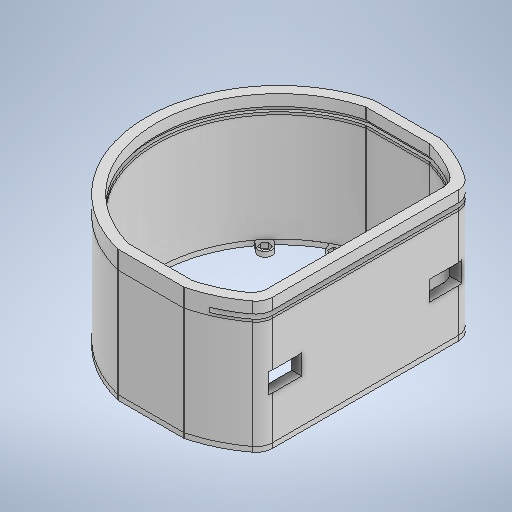
# Autodesk Inventor part: carcasa4.0
Saved by Autodesk Inventor 2025.3 (Build 293356030, 356C)
## iProperties
Created: 2025-08-27
Part Number: carcasa4.0
Material: Generic
Document SubType Name: Modeling
Designer: cdavi
Density: 1 g/cm^3
Appearance: Default
Author: cdavi
Autodesk Inventor part; units mm, degrees
ref_plane "YZ Plane" through (0, 0, 0) normal (1, 0, 0) x (0, 1, 0)
ref_plane "XZ Plane" through (0, 0, 0) normal (0, 1, 0) x (-1, 0, 0)
ref_plane "XY Plane" through (0, 0, 0) normal (0, 0, 1) x (1, 0, 0)
sketch "Sketch1" plane through (0, 0, 0) normal (0, 1, 0) x (-1, 0, 0)
  line L0 (18.8082, 71.5) -> (-18.8082, 71.5)
  line L1 (0, 0) -> (-52, 0) construction
  line L2 (19.5895, 77.5) -> (-19.5895, 77.5)
  line L3 (18.8082, -71.5) -> (-19.0722, -71.5)
  line L4 (19.5895, -77.5) -> (-19.5895, -77.5)
  line L5 (0, 0) -> (0, 77.5) construction
  line L6 (-46, 52.915) -> (-46, -52.915)
  line L7 (-52, 56) -> (-52, -56)
  arc A0 (-41.625, -61.183) -> (-19.0722, -71.5) centre (0, 0) ccw
  arc A1 (-48, -64) -> (-20.0918, -77.4359) centre (0, 0) ccw
  arc A2 (20.0918, -77.4359) -> (20.0918, 77.4359) centre (0, 0) ccw
  arc A3 (-20.0918, 77.4359) -> (-48, 64) centre (0, 0) ccw
  arc A4 (19.3307, -71.4306) -> (19.3307, 71.4306) centre (0, 0) ccw
  arc A5 (-19.3307, 71.4306) -> (-41.625, 61.183) centre (0, 0) ccw
  arc A6 (-20.0918, -77.4359) -> (-19.5895, -77.5) centre (-19.5895, -75.5) ccw
  arc A7 (19.5895, -77.5) -> (20.0918, -77.4359) centre (19.5895, -75.5) ccw
  arc A8 (18.8082, -71.5) -> (19.3307, -71.4306) centre (18.8082, -69.5) ccw
  arc A9 (19.3307, 71.4306) -> (18.8082, 71.5) centre (18.8082, 69.5) ccw
  arc A10 (20.0918, 77.4359) -> (19.5895, 77.5) centre (19.5895, 75.5) ccw
  arc A11 (-18.8082, 71.5) -> (-19.3307, 71.4306) centre (-18.8082, 69.5) ccw
  arc A12 (-19.5895, 77.5) -> (-20.0918, 77.4359) centre (-19.5895, 75.5) ccw
  arc A13 (-41.625, 61.183) -> (-46, 52.915) centre (-36, 52.915) ccw
  arc A14 (-48, 64) -> (-52, 56) centre (-42, 56) ccw
  arc A15 (-52, -56) -> (-48, -64) centre (-42, -56) ccw
  arc A16 (-46, -52.915) -> (-41.625, -61.183) centre (-36, -52.915) ccw
  point P0 (-19.8431, 77.5)
  point P1 (19.0722, -71.5)
  point P2 (19.8431, -77.5)
  point P3 (-19.8431, -77.5)
  point P4 (-52, -60.7947)
  point P5 (-46, 57.9655)
  point P6 (-46, -57.9655)
  point P7 (-52, 60.7947)
  point P8 (19.8431, 77.5)
  point P9 (19.0722, 71.5)
  point P10 (-19.0722, 71.5)
  dimension "d2" = 71.5
  dimension "d4" = 6
  dimension "d6" = 46
  dimension "d7" = 6
  dimension "d8" = 2
  dimension "d9" = 10
  dimension "d10" = 74
  dimension "d11" = 80
  dimension "d12" = 74
  dimension "d13" = 80
  constraints: 45 point on circle, 22 tangent, 17 centre point, 16 end point, 11 point on line, 9 equal radius, 4 symmetric about line, 3 vertical, 2 coincident, 2 horizontal, 2 midpoint, 1 parallel
  measures "d2" distance between parallel lines of L1 L0
  measures "d4" distance between parallel lines of L0 L2
  measures "d6" distance between parallel lines of L6 L5
  measures "d7" distance between parallel lines of L7 L6
  measures "d8" radius of A6
  measures "d9" radius of A13
  measures "d10" radius of A4
  measures "d11" radius of A2
  measures "d12" radius of A0
  measures "d13" radius of A1
extrude "Extrusion1" add sketch "Sketch1" along normal blind 65
sketch "Sketch2" plane through (52, 0, 56) normal (1, 0, 0) x (0, 0, -1)
  line L0 (56, 0) -> (56, 65) construction
  line L1 (108.915, 65) -> (3.085, 65) projected
  line L2 (-2.4359, 38) -> (17.5641, 38)
  line L3 (17.5641, 38) -> (17.5641, 26)
  line L4 (17.5641, 26) -> (-2.4359, 26)
  line L5 (-2.4359, 26) -> (-2.4359, 38)
  line L6 (0, 0) -> (112, 0) projected
  line L7 (-21.4359, 0) -> (-21.4359, 65) projected
  line L8 (114.4359, 38) -> (94.4359, 38)
  line L9 (94.4359, 38) -> (94.4359, 26)
  line L10 (94.4359, 26) -> (114.4359, 26)
  line L11 (114.4359, 26) -> (114.4359, 38)
  dimension "d16" = 26
  dimension "d17" = 19
  dimension "d18" = 12
  dimension "d19" = 20
  constraints: 18 end point, 4 symmetric about line, 2 parallel, 1 horizontal, 1 midpoint, 1 perpendicular
  measures "d16" distance between parallel lines of L6 L4
  measures "d17" distance between parallel lines of L5 L7
  measures "d18" distance of L2.end L3.end
  measures "d19" distance of L2.start L2.end
extrude "Extrusion2" cut sketch "Sketch2" against normal blind 13.25
sketch "Sketch3" plane through (52, 0, 56) normal (1, 0, 0) x (0, 0, -1)
  line L0 (3.568, 49.2223) -> (17.7975, 43.9952) construction
  line L1 (2.8909, 47.379) -> (17.1204, 42.1519)
  line L2 (18.4746, 45.8385) -> (4.2452, 51.0656)
  arc A0 (4.2452, 51.0656) -> (2.8909, 47.379) centre (3.568, 49.2223) ccw
  arc A1 (17.1204, 42.1519) -> (18.4746, 45.8385) centre (17.7975, 43.9952) ccw
  arc A2 (44.4296, 11.624) -> (34.6921, 2.9774) centre (43.8866, 2.4292) ccw construction
  arc A3 (44.531, 13.3402) -> (32.9759, 3.0797) centre (43.8866, 2.4292) ccw
  arc A4 (44.3283, 9.9077) -> (36.4083, 2.8751) centre (43.8866, 2.4292) ccw
  arc A5 (44.3283, 9.9077) -> (44.531, 13.3402) centre (44.4296, 11.624) ccw
  arc A6 (32.9759, 3.0797) -> (36.4083, 2.8751) centre (34.6921, 2.9774) ccw
  line L3 (56, 0) -> (56, 65) construction
  line L4 (109.1091, 47.379) -> (94.8796, 42.1519)
  line L5 (93.5254, 45.8385) -> (107.7548, 51.0656)
  arc A7 (109.1091, 47.379) -> (107.7548, 51.0656) centre (108.432, 49.2223) ccw
  arc A8 (93.5254, 45.8385) -> (94.8796, 42.1519) centre (94.2025, 43.9952) ccw
  point P0 (10.6828, 46.6088)
  constraints: 18 point on circle, 12 end point, 9 centre point, 8 tangent, 6 symmetric about line, 1 midpoint, 1 parallel, 2 other
extrude "Extrusion3" [suppressed]
extrude "Extrusion4" add sketch "Sketch1" along normal blind 3 from surface at 65 separate body contours A9 A4 A8 L3 A0 A16 L6 A13 A5 A11 L0 | A10 A2 A7 L4 A6 A1 A15 L7 A14 A3 A12 L2
sketch "Sketch5" plane through (-19.5895, 68, 77.5) normal (0, 1, 0) x (1, 0, 0)
  circle A0 centre (19.5895, 77.5) radius 8.5
  circle A1 centre (-10.4105, 77.5) radius 2.5
  line L0 (27.7136, 75) -> (36.5895, 75)
  line L1 (36.5895, 75) -> (36.5895, 80)
  line L2 (36.5895, 80) -> (27.7136, 80)
  line L3 (36.5895, 77.5) -> (71.5895, 77.5)
  line L4 (71.5895, 21.5) -> (71.5895, 133.5) projected
  line L5 (-10.4105, 77.5) -> (-60.4105, 77.5)
  arc A2 (-0.5023, 154.9359) -> (-0.5023, 0.0641) centre (19.5895, 77.5) ccw projected
  dimension "d26" = 17
  dimension "d27" = 5
  dimension "d31" = 5
  dimension "d32" = 17
  dimension "d47" = 30
  dimension "d204" = 35
  dimension "d205" = 50
  dimension "d206" = 52
  constraints: 10 end point, 3 point on circle, 2 centre point, 2 horizontal alignment, 2 midpoint, 2 perpendicular, 1 coincident, 1 horizontal, 1 point on line
  measures "d26" diameter of A0
  measures "d27" diameter of A1
  measures "d31" distance between parallel lines of L2 L0
  measures "d32" distance from line of A0.centre L1
  measures "d47" distance of A0.centre L5.start
  measures "d204" distance of L3.start L3.end
  measures "d205" distance of L5.start L5.end
  measures "d206" distance from line of L4 point (19.59, 77.5)
extrude "Extrusion5" cut sketch "Sketch5" against normal through all bodies 2
sketch "Sketch6" plane through (0, 0, 0) normal (0, 1, 0) x (-1, 0, 0)
  circle A0 centre (0, 0) radius 69 construction
  arc A1 (-19.3307, 71.4306) -> (-41.625, 61.183) centre (0, 0) ccw projected
  arc A2 (-41.625, 61.183) -> (-46, 52.915) centre (-36, 52.915) ccw projected
  line L0 (-46, -52.915) -> (-46, 52.915) projected
  arc A3 (-46, -52.915) -> (-41.625, -61.183) centre (-36, -52.915) ccw projected
  arc A4 (-41.625, -61.183) -> (-19.0722, -71.5) centre (0, 0) ccw projected
  line L1 (18.8082, -71.5) -> (-19.0722, -71.5) construction
  arc A5 (19.3307, -71.4306) -> (19.3307, 71.4306) centre (0, 0) ccw projected
  line L2 (-18.8082, 71.5) -> (18.8082, 71.5) construction
  line L3 (19.5895, 77.5) -> (-19.5895, 77.5) projected
  arc A6 (-20.0918, 77.4359) -> (-48, 64) centre (0, 0) ccw projected
  arc A7 (-48, 64) -> (-52, 56) centre (-42, 56) ccw projected
  line L4 (-52, 56) -> (-52, -56) projected
  arc A8 (-52, -56) -> (-48, -64) centre (-42, -56) ccw projected
  arc A9 (-48, -64) -> (-20.0918, -77.4359) centre (0, 0) ccw projected
  line L5 (-19.5895, -77.5) -> (19.5895, -77.5) projected
  arc A10 (20.0918, -77.4359) -> (20.0918, 77.4359) centre (0, 0) ccw projected
  arc A11 (-18.5383, 65.4242) -> (-38.25, 56.2222) centre (0, 0) ccw construction
  arc A12 (-38.25, 56.2222) -> (-40, 52.915) centre (-36, 52.915) ccw construction
  line L6 (-40, 52.915) -> (-40, -52.915) construction
  arc A13 (-40, -52.915) -> (-38.25, -56.2222) centre (-36, -52.915) ccw construction
  arc A14 (-38.25, -56.2222) -> (-18.5383, -65.4242) centre (0, 0) ccw construction
  line L7 (-17.9931, -65.5) -> (17.9931, -65.5) construction
  line L8 (-17.9931, 65.5) -> (17.9931, 65.5) construction
  arc A15 (18.5383, -65.4242) -> (18.5383, 65.4242) centre (0, 0) ccw construction
  arc A16 (-8.124, -2.5) -> (-8.124, 2.5) centre (0, 0) ccw projected
  line L9 (0, 0) -> (52.8571, 44.3523) construction
  line L10 (0, 0) -> (80, 0) construction
  circle A17 centre (52.8571, 44.3523) radius 3.1 construction
  line L11 (0, 0) -> (0, -69) construction
  circle A18 centre (29.1607, 62.5352) radius 3.1 construction
  line L12 (29.1607, 62.5352) -> (0, 0) construction
  circle A19 centre (-42.5, 20) radius 3.1 construction
  circle A20 centre (-29.1607, 62.5352) radius 3.1 construction
  line L13 (-29.1607, 62.5352) -> (0, 0) construction
  arc A21 (-17.9931, 65.5) -> (-18.5383, 65.4242) centre (-17.9931, 63.5) ccw construction
  arc A22 (-18.5383, -65.4242) -> (-17.9931, -65.5) centre (-17.9931, -63.5) ccw construction
  arc A23 (17.9931, -65.5) -> (18.5383, -65.4242) centre (17.9931, -63.5) ccw construction
  arc A24 (18.5383, 65.4242) -> (17.9931, 65.5) centre (17.9931, 63.5) ccw construction
  arc A25 (-20.0918, -77.4359) -> (-19.5895, -77.5) centre (-19.5895, -75.5) ccw projected
  arc A26 (19.5895, -77.5) -> (20.0918, -77.4359) centre (19.5895, -75.5) ccw projected
  arc A27 (20.0918, 77.4359) -> (19.5895, 77.5) centre (19.5895, 75.5) ccw projected
  arc A28 (-19.5895, 77.5) -> (-20.0918, 77.4359) centre (-19.5895, 75.5) ccw projected
  circle A29 centre (52.8571, -44.3523) radius 3.1 construction
  circle A30 centre (29.1607, -62.5352) radius 3.1 construction
  circle A31 centre (-42.5, -20) radius 3.1 construction
  circle A32 centre (-29.1607, -62.5352) radius 3.1 construction
  line L14 (19.3307, 65.1945) -> (19.3307, 71.4306)
  line L15 (-19.3307, 65.1945) -> (-19.3307, 71.4306)
  line L16 (19.3307, 71.4306) -> (-19.3307, 71.4306)
  line L17 (19.3307, -65.1945) -> (19.3307, -71.4306)
  line L18 (-19.3307, -65.1945) -> (-19.3307, -71.4306)
  line L19 (19.3307, -71.4306) -> (-19.3307, -71.4306)
  circle A33 centre (52.8571, 44.3523) radius 4
  circle A34 centre (29.1607, 62.5352) radius 4
  line L20 (49.8042, 43.814) -> (50.8644, 46.7271)
  line L21 (50.8644, 46.7271) -> (53.9173, 47.2654)
  line L22 (53.9173, 47.2654) -> (55.91, 44.8907)
  line L23 (55.91, 44.8907) -> (54.8497, 41.9776)
  line L24 (54.8497, 41.9776) -> (51.7968, 41.4393)
  line L25 (51.7968, 41.4393) -> (49.8042, 43.814)
  line L26 (26.6213, 60.7572) -> (26.3511, 63.8454)
  line L27 (26.3511, 63.8454) -> (28.8905, 65.6234)
  line L28 (28.8905, 65.6234) -> (31.7, 64.3133)
  line L29 (31.7, 64.3133) -> (31.9702, 61.2251)
  line L30 (31.9702, 61.2251) -> (29.4308, 59.447)
  line L31 (29.4308, 59.447) -> (26.6213, 60.7572)
  circle A35 centre (-42.5, 20) radius 4
  line L32 (-45.1847, 18.45) -> (-45.1847, 21.55)
  line L33 (-45.1847, 21.55) -> (-42.5, 23.1)
  line L34 (-42.5, 23.1) -> (-39.8153, 21.55)
  line L35 (-39.8153, 21.55) -> (-39.8153, 18.45)
  line L36 (-39.8153, 18.45) -> (-42.5, 16.9)
  line L37 (-42.5, 16.9) -> (-45.1847, 18.45)
  line L38 (-42.5, 24) -> (-46, 24)
  line L39 (-42.5, 16) -> (-46, 16)
  circle A36 centre (-29.1607, 62.5352) radius 4
  line L40 (-29.4308, 59.447) -> (-31.9702, 61.2251)
  line L41 (-31.9702, 61.2251) -> (-31.7, 64.3133)
  line L42 (-31.7, 64.3133) -> (-28.8905, 65.6234)
  line L43 (-28.8905, 65.6234) -> (-26.3511, 63.8454)
  line L44 (-26.3511, 63.8454) -> (-26.6213, 60.7572)
  line L45 (-26.6213, 60.7572) -> (-29.4308, 59.447)
  line L46 (-32.7354, 60.7404) -> (-34.9798, 65.2105)
  circle A37 centre (52.8571, -44.3523) radius 4
  circle A38 centre (29.1607, -62.5352) radius 4
  circle A39 centre (-42.5, -20) radius 4
  line L47 (-42.5, -24) -> (-46, -24)
  line L48 (-42.5, -16) -> (-46, -16)
  circle A40 centre (-29.1607, -62.5352) radius 4
  line L49 (-32.7354, -60.7404) -> (-34.9798, -65.2105)
  line L50 (49.8042, -43.814) -> (50.8644, -46.7271)
  line L51 (50.8644, -46.7271) -> (53.9173, -47.2654)
  line L52 (53.9173, -47.2654) -> (55.91, -44.8907)
  line L53 (55.91, -44.8907) -> (54.8497, -41.9776)
  line L54 (54.8497, -41.9776) -> (51.7968, -41.4393)
  line L55 (51.7968, -41.4393) -> (49.8042, -43.814)
  line L56 (26.6213, -60.7572) -> (26.3511, -63.8454)
  line L57 (26.3511, -63.8454) -> (28.8905, -65.6234)
  line L58 (28.8905, -65.6234) -> (31.7, -64.3133)
  line L59 (31.7, -64.3133) -> (31.9702, -61.2251)
  line L60 (31.9702, -61.2251) -> (29.4308, -59.447)
  line L61 (29.4308, -59.447) -> (26.6213, -60.7572)
  line L62 (-29.4308, -59.447) -> (-31.9702, -61.2251)
  line L63 (-31.9702, -61.2251) -> (-31.7, -64.3133)
  line L64 (-31.7, -64.3133) -> (-28.8905, -65.6234)
  line L65 (-28.8905, -65.6234) -> (-26.3511, -63.8454)
  line L66 (-26.3511, -63.8454) -> (-26.6213, -60.7572)
  line L67 (-26.6213, -60.7572) -> (-29.4308, -59.447)
  line L68 (-45.1847, -18.45) -> (-45.1847, -21.55)
  line L69 (-45.1847, -21.55) -> (-42.5, -23.1)
  line L70 (-42.5, -23.1) -> (-39.8153, -21.55)
  line L71 (-39.8153, -21.55) -> (-39.8153, -18.45)
  line L72 (-39.8153, -18.45) -> (-42.5, -16.9)
  line L73 (-42.5, -16.9) -> (-45.1847, -18.45)
  line L74 (50.1982, 47.3407) -> (53.9351, 50.6656)
  line L75 (55.3383, 41.2149) -> (59.2616, 44.3177)
  line L76 (32.7354, 60.7404) -> (34.9798, 65.2105)
  line L77 (50.1982, -47.3407) -> (53.9351, -50.6656)
  line L78 (55.3383, -41.2149) -> (59.2616, -44.3177)
  line L79 (32.7354, -60.7404) -> (34.9798, -65.2105)
  line L80 (-25.488, 64.1199) -> (-27.4696, 68.7126)
  line L81 (25.488, 64.1199) -> (27.4696, 68.7126)
  line L82 (-25.488, -64.1199) -> (-27.4696, -68.7126)
  line L83 (25.488, -64.1199) -> (27.4696, -68.7126)
  line L84 (-18.8082, 71.5) -> (-52, 71.5)
  line L85 (-52, 71.5) -> (-52, 56)
  line L86 (-35.8852, 71.5) -> (-18.8082, 71.5)
  point P0 (-18.2688, -65.5)
  point P1 (-19.3307, 65.1945)
  point P2 (-19.3307, -65.1945)
  point P3 (29.1607, 62.5352)
  point P4 (-19.3307, -71.4306)
  point P5 (-34.9798, -65.2105)
  point P6 (-46, -24)
  point P7 (-46, -16)
  point P8 (59.2616, -44.3177)
  point P9 (55.3383, -41.2149)
  point P10 (34.9798, -65.2105)
  point P11 (-27.9581, 66.3502)
  point P12 (-27.9581, -66.3502)
  point P13 (27.9581, -66.3502)
  point P14 (27.9581, 66.3502)
  point P15 (-46, 21.9365)
  point P16 (-46, 18.0635)
  point P17 (-32.8561, 64.0662)
  point P18 (32.8561, -64.0662)
  point P19 (56.8533, -44.1781)
  point P20 (53.3794, -48.3181)
  point P21 (-32.8561, -64.0662)
  point P22 (-46, -21.9365)
  point P23 (-46, -18.0635)
  point P24 (53.3794, 48.3181)
  point P25 (56.8533, 44.1781)
  point P26 (32.8561, 64.0662)
  point P27 (25.488, -64.1199)
  point P28 (27.4696, -68.7126)
  point P29 (-25.488, -64.1199)
  point P30 (34.0084, -67.0387)
  point P31 (-28.5882, -71.3052)
  point P32 (28.5882, -71.3052)
  point P33 (28.5882, 71.3052)
  point P34 (-28.5882, 71.3052)
  point P35 (34.0084, 67.0387)
  point P36 (-19.3307, -71.4306)
  point P37 (-34.0084, -67.0387)
  point P38 (-34.0084, 67.0387)
  dimension "d33" = 138
  dimension "d39" = 6.2
  dimension "d34" = 6
  dimension "d35" = 6
  dimension "d36" = 6
  dimension "d37" = 40
  dimension "d38" = 25
  dimension "d40" = 20
  dimension "d41" = 3.5
  dimension "d42" = 25
  dimension "d44" = 2
  dimension "d61" = 8
  dimension "d62" = 8
  dimension "d63" = 8
  dimension "d64" = 8
  dimension "d171" = 90
  dimension "d172" = 15.5
  constraints: 162 end point, 52 symmetric about line, 38 point on circle, 20 centre point, 16 tangent, 10 coincident, 6 perpendicular, 4 point on line, 3 equal radius, 2 parallel, 2 vertical, 1 collinear, 1 horizontal, 93 other
  measures "d34" radial gap between concentric circles of A1 A11
  measures "d35" distance between parallel lines of L2 L8
  measures "d36" radial gap between concentric circles of A5 A15
  measures "d37" angle of L10 L9
  measures "d38" angle of L11 L12
  measures "d40" distance from line of point (-42.5, 20) L10
  measures "d41" distance from line of L0 point (-42.5, 20)
  measures "d42" angle of L11 L13
  measures "d44" radius of A21
  measures "d61" diameter of A33
  measures "d62" diameter of A34
  measures "d63" diameter of A35
  measures "d64" diameter of A36
  measures "d171" angle of L85 L84
  measures "d172" distance of L84.end L4.start
extrude "Extrusion6" add sketch "Sketch6" against normal blind 3 separate body contours L80 A36 L46 A1 | A36 | A5 L76 A34 L81 | A34 | A5 L75 A33 L74 | L38 A35 L0 | A33 | A35 L0 | L0 A35 | A5 L77 A37 L78 | A35 L39 L0 | A37 | A5 L83 A38 L79 | L48 A39 L0 | A38 | A39 L0 | L0 A39 | A39 L47 L0 | A4 L49 A40 L82 | A40 | A27 A10 A26 L5 A25 A9 A8 L4 A7 A6 A28 L3
sketch "Sketch14" plane through (0, 65, 0) normal (0, 1, 0) x (1, 0, 0)
  arc A0 (-20.0918, 77.4359) -> (-20.0918, -77.4359) centre (0, 0) ccw projected
  arc A1 (-20.0918, -77.4359) -> (-19.5895, -77.5) centre (-19.5895, -75.5) ccw projected
  line L0 (-19.5895, -77.5) -> (19.5895, -77.5) projected
  arc A2 (19.5895, -77.5) -> (20.0918, -77.4359) centre (19.5895, -75.5) ccw projected
  arc A3 (20.0918, -77.4359) -> (48, -64) centre (0, 0) ccw projected
  arc A4 (48, -64) -> (52, -56) centre (42, -56) ccw projected
  line L1 (52, -56) -> (52, 56) projected
  arc A5 (52, 56) -> (48, 64) centre (42, 56) ccw projected
  arc A6 (48, 64) -> (20.0918, 77.4359) centre (0, 0) ccw projected
  arc A7 (20.0918, 77.4359) -> (19.5895, 77.5) centre (19.5895, 75.5) ccw projected
  line L2 (19.5895, 77.5) -> (-19.5895, 77.5) projected
  arc A8 (-19.5895, 77.5) -> (-20.0918, 77.4359) centre (-19.5895, 75.5) ccw projected
  line L3 (-18.8082, 71.5) -> (19.0722, 71.5) projected
  arc A9 (41.625, 61.183) -> (19.0722, 71.5) centre (0, 0) ccw projected
  arc A10 (46, 52.915) -> (41.625, 61.183) centre (36, 52.915) ccw projected
  line L4 (46, 52.915) -> (46, -52.915) projected
  arc A11 (41.625, -61.183) -> (46, -52.915) centre (36, -52.915) ccw projected
  arc A12 (19.3307, -71.4306) -> (41.625, -61.183) centre (0, 0) ccw projected
  arc A13 (18.8082, -71.5) -> (19.3307, -71.4306) centre (18.8082, -69.5) ccw projected
  line L5 (18.8082, -71.5) -> (-18.8082, -71.5) projected
  arc A14 (-19.3307, -71.4306) -> (-18.8082, -71.5) centre (-18.8082, -69.5) ccw projected
  arc A15 (-19.3307, 71.4306) -> (-19.3307, -71.4306) centre (0, 0) ccw projected
  arc A16 (-18.8082, 71.5) -> (-19.3307, 71.4306) centre (-18.8082, 69.5) ccw projected
extrude "Extrusion11" add sketch "Sketch14" along normal blind 6 separate body
sketch "Sketch15" plane through (52, 65, 56) normal (1, 0, 0) x (0, 0, -1)
  line L0 (56, 6) -> (56, 0)
  line L1 (56, 6) -> (0, 6)
  line L2 (0, 6) -> (-17.5, 6)
  line L3 (-17.5, 6) -> (-17.5, 0)
  line L4 (-17.5, 0) -> (0, 0)
  line L5 (0, 0) -> (56, 0)
  line L6 (3.085, 0) -> (56, 0)
  line L7 (56, 6) -> (0, 6)
  line L8 (56, 6) -> (56, 4.5)
  line L9 (56, 4.5) -> (0, 4.246)
  line L10 (0, 0) -> (0, 6) projected
  line L11 (56, 0) -> (56, 1.5)
  line L12 (56, 1.5) -> (0, 1.5)
  arc A0 (56, 4.5) -> (56, 4.5) centre (55.2781, 163.6578) ccw
  line L13 (0, 4.246) -> (-17.5, 4.246)
  line L14 (0, 1.5) -> (-17.5, 1.5)
  line L15 (56, 6) -> (112, 6)
  line L16 (112, 6) -> (129.5, 6)
  line L17 (129.5, 6) -> (129.5, 0)
  line L18 (129.5, 0) -> (112, 0)
  line L19 (112, 0) -> (56, 0)
  line L20 (108.915, 0) -> (56, 0)
  line L21 (56, 6) -> (112, 6)
  line L22 (56, 4.5) -> (112, 4.246)
  line L23 (112, 0) -> (112, 6)
  line L24 (56, 1.5) -> (112, 1.5)
  arc A1 (56, 4.5) -> (56, 4.5) centre (56.7219, 163.6578) ccw
  line L25 (112, 4.246) -> (129.5, 4.246)
  line L26 (112, 1.5) -> (129.5, 1.5)
  point P0 (56, -65)
  dimension "d173" = 17.5
  dimension "d176" = 1.5
  dimension "d177" = 1.5
  dimension "d202" = 2.746
  constraints: 52 end point, 15 point on line, 11 symmetric about line, 6 perpendicular, 4 point on circle, 2 centre point, 1 collinear, 1 tangent, 1 other
  measures "d173" distance of L1.end L2.end
  measures "d176" distance of L0.start L8.end
  measures "d177" distance of L0.end L11.end
  measures "d202" distance between parallel lines of L14 L13
extrude "Extrusion12" cut sketch "Sketch15" against normal blind 71.33 contours L22 L23 L24 L0 | L0 L12 L10 L9 | L10 L14 L3 L13 | L25 L17 L26 L23 bodies 4
ref_plane "Work Plane1" through (0, 66.5, 0) normal (0, -1, 0) x (1, 0, 0)
sketch "Sketch18" plane through (0, 66.5, 0) normal (0, -1, 0) x (1, 0, 0)
  line L0 (52, 56) -> (52, -56) projected
  line L1 (52, 0) -> (-80, 0)
  arc A0 (-20.0918, 77.4359) -> (-20.0918, -77.4359) centre (0, 0) ccw projected
  arc A1 (-80, 0) -> (-20.0918, -77.4359) centre (0, 0) ccw
  arc A2 (-74, 0) -> (-19.33, -71.4307) centre (0, 0) ccw
  arc A3 (-76, 0) -> (-19.33, -73.5007) centre (0, 0) ccw
  arc A4 (-19.33, -71.4307) -> (-18.8082, -71.5) centre (-18.8082, -69.5) ccw projected
  line L2 (-19.33, -71.4307) -> (-19.33, -73.5)
  arc A5 (-19.33, 71.4307) -> (-74, 0) centre (0, 0) ccw
  arc A6 (-19.33, 73.5007) -> (-76, 0) centre (0, 0) ccw
  line L3 (-19.33, 71.4307) -> (-19.33, 73.5)
  line L4 (-19.33, -73.5007) -> (-19.33, -71.4307)
  line L5 (-19.33, 73.5007) -> (-19.33, 71.4307)
  point P0 (19.0722, -71.5)
  point P1 (-19.5585, 71.3685)
  point P2 (-19.5585, -71.3685)
  point P3 (-18.8082, 71.5)
  point P4 (-19.5585, -71.3685)
  point P5 (-20.0918, 77.4359)
  point P6 (-18.8082, -73.6359)
  point P7 (-18.8082, 73.6359)
  point P8 (-18.8082, 73.6359)
  constraints: 12 point on circle, 10 end point, 7 symmetric about line, 6 point on line, 5 centre point, 3 coincident, 1 collinear, 1 horizontal, 1 midpoint, 1 vertical, 3 other
extrude "Extrusion14" cut sketch "Sketch18" against normal blind 2.746 bodies 4
sketch "Sketch19" plane through (0, 71, 0) normal (0, 1, 0) x (1, 0, 0)
  line L0 (18.8082, -71.5) -> (-18.8082, -71.5) projected
  line L1 (-19.5895, -77.5) -> (19.5895, -77.5) projected
  arc A0 (18.8082, -71.5) -> (19.3307, -71.4306) centre (18.8082, -69.5) ccw projected
  arc A1 (20.0918, -77.4359) -> (48, -64) centre (0, 0) ccw projected
  arc A2 (19.5895, -77.5) -> (20.0918, -77.4359) centre (19.5895, -75.5) ccw projected
  arc A3 (19.3307, -71.4306) -> (41.625, -61.183) centre (0, 0) ccw projected
  arc A4 (48, -64) -> (52, -56) centre (42, -56) ccw projected
  arc A5 (41.625, -61.183) -> (46, -52.915) centre (36, -52.915) ccw projected
  line L2 (46, 52.915) -> (46, -52.915) projected
  line L3 (52, -56) -> (52, 56) projected
  arc A6 (52, 56) -> (48, 64) centre (42, 56) ccw projected
  arc A7 (46, 52.915) -> (41.625, 61.183) centre (36, 52.915) ccw projected
  arc A8 (48, 64) -> (20.0918, 77.4359) centre (0, 0) ccw projected
  arc A9 (41.625, 61.183) -> (19.0722, 71.5) centre (0, 0) ccw projected
  line L4 (-18.8082, 71.5) -> (19.0722, 71.5) projected
  arc A10 (20.0918, 77.4359) -> (19.5895, 77.5) centre (19.5895, 75.5) ccw projected
  line L5 (19.5895, 77.5) -> (-19.5895, 77.5) projected
  arc A11 (-19.5895, 77.5) -> (-20.0918, 77.4359) centre (-19.5895, 75.5) ccw projected
  arc A12 (-18.8082, 71.5) -> (-19.3307, 71.4306) centre (-18.8082, 69.5) ccw projected
  arc A13 (-19.3307, 71.4306) -> (-19.3307, -71.4306) centre (0, 0) ccw projected
  arc A14 (-20.0918, 77.4359) -> (-20.0918, -77.4359) centre (0, 0) ccw projected
  arc A15 (-19.3307, -71.4306) -> (-18.8082, -71.5) centre (-18.8082, -69.5) ccw projected
  arc A16 (-20.0918, -77.4359) -> (-19.5895, -77.5) centre (-19.5895, -75.5) ccw projected
extrude "Extrusion15" add sketch "Sketch19" along normal blind 5 bodies 4
body "Solid1"
body "Solid2"
body "Solid3"
body "Solid4"
